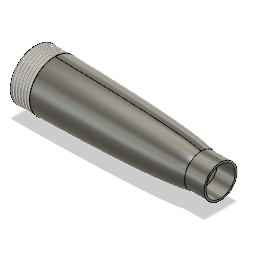
nose02 (Autodesk Fusion 360 design; units mm, degrees)
Autodesk Fusion 360 part; units mm, degrees
sketch "スケッチ1" plane through (0, 0, 0) normal (0, 0, 1) x (1, 0, 0)
sketch "スケッチ2" plane through (0, 0, 0) normal (0, 0, 1) x (1, 0, 0)
sketch "スケッチ3" plane through (0, 0, 0) normal (0, 0, 1) x (1, 0, 0)
sketch "スケッチ4" plane through (0, 0, 0) normal (1, 0, 0) x (0, 0, -1)
sketch "スケッチ5" plane through (0, 0, 0) normal (0, 0, 1) x (1, 0, 0)
sketch "スケッチ6" plane through (0, 0, 0) normal (0, 0, 1) x (1, 0, 0)
sketch "スケッチ7" plane through (0, 0, 0) normal (0, 0, 1) x (1, 0, 0)
  line L0 (85, 0) -> (86, 0)
  line L1 (86, 0) -> (86, 7.5)
  line L2 (86, 7.5) -> (95, 7.5)
  line L3 (95, 7.5) -> (95, 9.1)
  line L4 (95, 9.1) -> (85, 9.1)
  line L5 (85, 9.1) -> (85, 0)
  line L6 (85, 9.1) -> (85, 7.5)
sketch "スケッチ8" plane through (0, 0, 0) normal (0, 0, 1) x (1, 0, 0)
  line L0 (85, 0) -> (86, 0)
  line L1 (85, 7.5) -> (85, 0)
sketch "スケッチ9" plane through (0, 0, 0) normal (0, 0, 1) x (1, 0, 0)
  line L0 (10, 13.6) -> (10, 12.8)
  line L1 (10, 12.8) -> (0, 12.8)
  line L2 (0, 12.8) -> (0, 12)
  line L3 (0, 12) -> (10, 12)
  line L4 (10, 12.8) -> (0, 12.8)
  line L5 (0, 12) -> (10, 12)
  line L6 (10, 12) -> (10, 13.6)
sketch "スケッチ10" plane through (0, 0, 0) normal (0, 0, 1) x (1, 0, 0)
  spline S0 degree 2 poles (10, 13.6) (73.6996, 13.2) (85, 9.1) knots 0 0 0 7.522305 7.522305 7.522305
sketch "スケッチ11" plane through (0, 0, 0) normal (0, 0, 1) x (1, 0, 0)
  line L0 (0, 12.8) -> (0, 12)
sketch "スケッチ12" plane through (0, 0, 0) normal (0, 0, 1) x (1, 0, 0)
sketch "スケッチ13" plane through (0, 0, 0) normal (0, 0, 1) x (1, 0, 0)
  spline S0 degree 2 poles (10, 12) (73.7004, 10.892) (85, 7.5) knots 0 0 0 7.519038 7.519038 7.519038
sketch "スケッチ14" plane through (0, 0, 0) normal (0, 0, 1) x (1, 0, 0)
  spline S0 degree 2 poles (10, 13.6) (73.6996, 13.2) (85, 9.1) knots 0 0 0 7.522305 7.522305 7.522305
  spline S1 degree 2 poles (10, 12) (73.7004, 10.892) (85, 7.5) knots 0 0 0 7.519038 7.519038 7.519038
sketch "スケッチ15" plane through (0, 0, 0) normal (0, 0, 1) x (1, 0, 0)
sketch "スケッチ16" plane through (0, 0, 0) normal (0, 0, 1) x (1, 0, 0)
sketch "スケッチ17" plane through (0, 0, 0) normal (0, 0, 1) x (1, 0, 0)
  line L0 (10, 13.6) -> (10, 12)
sketch "スケッチ18" plane through (0, 0, 0) normal (0, 0, 1) x (1, 0, 0)
  line L0 (85, 9.1) -> (85, 7.5)
sketch "スケッチ19" plane through (0, 0, 0) normal (0, 0, 1) x (1, 0, 0)
  spline S0 degree 2 poles (10, 13.6) (73.6996, 13.2) (85, 9.1) knots 0 0 0 7.522305 7.522305 7.522305
  spline S1 degree 2 poles (10, 12) (73.7004, 10.892) (85, 7.5) knots 0 0 0 7.519038 7.519038 7.519038
  line L0 (85, 9.1) -> (85, 7.5)
  line L1 (10, 13.6) -> (10, 12)
  line L2 (10, 12) -> (10, 13)
  line L3 (85, 7.5) -> (85, 8.5)
  line L4 (73.7004, 10.892) -> (73.7004, 11.892)
  spline S2 degree 2 poles (10, 13) (73.7004, 11.892) (85, 8.5) knots 0 0 0 7.519038 7.519038 7.519038
  line L5 (85, 8.5) -> (95, 8.5)
  line L6 (95, 8.5) -> (95, 7.5)
  line L7 (95, 7.5) -> (86, 7.5)
  line L8 (86, 7.5) -> (86, 0)
  line L9 (86, 0) -> (85, 0)
  line L10 (85, 0) -> (85, 7.5)
  dimension "d3" = 1
  dimension "d4" = 1
  dimension "d5" = 1
revolve "回転3" add sketch "スケッチ19" sketch "スケッチ9" angle 360 about axis through (1.75, 0, 0) along (1, 0, 0) contours S1 L0 L1 L2 L3 S2 | L0 L3 L5 L6 L7 L8 L9 L10 of sketch 2
thread "ねじ2" "ISO Metric profile 26.0 M26x1.5 6g" major diameter 25.85 minor diameter 24.1319 pitch 1.5 angle 60 resizes the face on face at (6.6667, 12.7585, -1.03)
revolve "回転2" [suppressed]
revolve "回転1" [suppressed]
thread "ねじ1" [suppressed]
